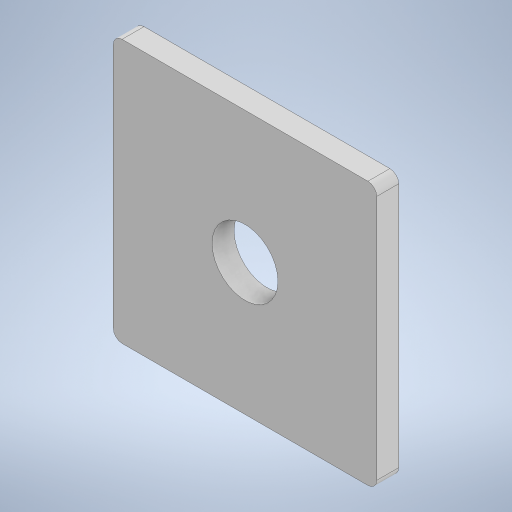
# Autodesk Inventor part: Motor clamp p1
Saved by Autodesk Inventor 2023 (Build 270158000, 158)
## iProperties
Created: 2022-06-04
Part Number: Motor clamp p1
Material: Generic
Document SubType Name: Modeling
Designer: prana_p9lsmih
Density: 1 g/cm^3
Appearance: Default
Author: prana_p9lsmih
Autodesk Inventor part; units mm, degrees
ref_plane "YZ Plane" through (0, 0, 0) normal (1, 0, 0) x (0, 1, 0)
ref_plane "XZ Plane" through (0, 0, 0) normal (0, 1, 0) x (-1, 0, 0)
ref_plane "XY Plane" through (0, 0, 0) normal (0, 0, 1) x (1, 0, 0)
sketch "Sketch1" plane through (0, 0, 0) normal (0, 0, 1) x (1, 0, 0)
  line L0 (0, 0) -> (60, 0)
  line L1 (60, 0) -> (60, 60)
  line L2 (60, 60) -> (0, 60)
  line L3 (0, 60) -> (0, 0)
  dimension "d0" = 60
  dimension "d1" = 60
  constraints: 8 end point, 3 perpendicular, 1 horizontal
  measures "d0" distance of L0.start L0.end
  measures "d1" distance of L0.end L1.end
extrude "Extrusion1" add sketch "Sketch1" along normal blind 5
sketch "Sketch2" plane through (0, 0, 5) normal (0, 0, 1) x (1, 0, 0)
  line L0 (60, 60) -> (0, 60) projected
  line L1 (60, 0) -> (60, 60) projected
  point P0 (0, 0)
  point P1 (30, 30)
  dimension "d4" = 30
  dimension "d5" = 30
  measures "d4" distance from line of L0 point (30, 30)
  measures "d5" distance from line of L1 point (30, 30)
hole "Hole1" at (30, 30, 5) direction (0, 0, -1) diameter 15 end through all
fillet "Fillet1" radius 2 4 edges at (60, 60, 2.5) (60, 0, 2.5) (0, 0, 2.5) (0, 60, 2.5)
sketch "Sketch5" plane through (0, 2, 0) normal (-1, 0, 0) x (0, 0, 1)
  line L0 (0, 56) -> (0, 0) projected
  line L1 (0, -2) -> (5, -2) projected
  point P0 (2.5, 33)
  dimension "d36" = 2.5
  dimension "d37" = 35
  measures "d36" distance from line of L0 point (2.5, 33)
  measures "d37" distance from line of L1 point (2.5, 33)
hole "Hole4" at (0, 35, 2.5) direction (1, 0, 0) diameter 2 depth 10 tip angle 118
body "Solid1"
